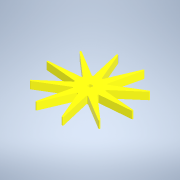
# Autodesk Inventor part: Star
Saved by Autodesk Inventor 2021 (Build 250183000, 183)
## iProperties
Created: 2021-05-22
Part Number: Star
Material: PC/ABS Plastic
Document SubType Name: Modeling
Designer: sami8
Density: 0.357273 g/cm^3
Appearance: Smooth - Yellow
Author: sami8
Autodesk Inventor part; units mm, degrees
ref_plane "YZ Plane" through (0, 0, 0) normal (1, 0, 0) x (0, 1, 0)
ref_plane "XZ Plane" through (0, 0, 0) normal (0, 1, 0) x (-1, 0, 0)
ref_plane "XY Plane" through (0, 0, 0) normal (0, 0, 1) x (1, 0, 0)
sketch "Sketch1" plane through (0, 0, 0) normal (0, 1, 0) x (-1, 0, 0)
  line L0 (2.4, -1.3856) -> (0, -2.7713)
  line L1 (0, -2.7713) -> (-2.4, -1.3856)
  line L2 (-2.4, -1.3856) -> (-2.4, 1.3856)
  line L3 (-2.4, 1.3856) -> (0, 2.7713)
  line L4 (0, 2.7713) -> (2.4, 1.3856)
  line L5 (2.4, 1.3856) -> (2.4, -1.3856)
  line L6 (0, 0) -> (2.4, 0) construction
  line L7 (0, 6) -> (70, 0)
  line L8 (70, 0) -> (0, -6)
  line L9 (0, 0) -> (0, -6)
  line L10 (0, 0) -> (0, 6)
  line L11 (0, 0) -> (70, 0) construction
  line L12 (-3.5267, 4.8541) -> (56.6312, 41.145)
  line L13 (0, 0) -> (-3.5267, 4.8541)
  line L14 (0, 0) -> (3.5267, -4.8541)
  line L15 (56.6312, 41.145) -> (3.5267, -4.8541)
  line L16 (-5.7063, 1.8541) -> (21.6312, 66.574)
  line L17 (0, 0) -> (-5.7063, 1.8541)
  line L18 (0, 0) -> (5.7063, -1.8541)
  line L19 (21.6312, 66.574) -> (5.7063, -1.8541)
  line L20 (-5.7063, -1.8541) -> (-21.6312, 66.574)
  line L21 (0, 0) -> (-5.7063, -1.8541)
  line L22 (0, 0) -> (5.7063, 1.8541)
  line L23 (-21.6312, 66.574) -> (5.7063, 1.8541)
  line L24 (-3.5267, -4.8541) -> (-56.6312, 41.145)
  line L25 (0, 0) -> (-3.5267, -4.8541)
  line L26 (0, 0) -> (3.5267, 4.8541)
  line L27 (-56.6312, 41.145) -> (3.5267, 4.8541)
  line L28 (0, -6) -> (-70, 0)
  line L29 (0, 0) -> (0, -6)
  line L30 (0, 0) -> (0, 6)
  line L31 (-70, 0) -> (0, 6)
  line L32 (3.5267, -4.8541) -> (-56.6312, -41.145)
  line L33 (0, 0) -> (3.5267, -4.8541)
  line L34 (0, 0) -> (-3.5267, 4.8541)
  line L35 (-56.6312, -41.145) -> (-3.5267, 4.8541)
  line L36 (5.7063, -1.8541) -> (-21.6312, -66.574)
  line L37 (0, 0) -> (5.7063, -1.8541)
  line L38 (0, 0) -> (-5.7063, 1.8541)
  line L39 (-21.6312, -66.574) -> (-5.7063, 1.8541)
  line L40 (5.7063, 1.8541) -> (21.6312, -66.574)
  line L41 (0, 0) -> (5.7063, 1.8541)
  line L42 (0, 0) -> (-5.7063, -1.8541)
  line L43 (21.6312, -66.574) -> (-5.7063, -1.8541)
  line L44 (3.5267, 4.8541) -> (56.6312, -41.145)
  line L45 (0, 0) -> (3.5267, 4.8541)
  line L46 (0, 0) -> (-3.5267, -4.8541)
  line L47 (56.6312, -41.145) -> (-3.5267, -4.8541)
  point P0 (14.6116, 4.7476)
  point P1 (9.0304, 12.4293)
  point P2 (0, 15.3635)
  point P3 (-9.0304, 12.4293)
  point P4 (-14.6116, 4.7476)
  point P5 (-14.6116, -4.7476)
  point P6 (-9.0304, -12.4293)
  point P7 (0, -15.3635)
  point P8 (9.0304, -12.4293)
  point P9 (14.6116, -4.7476)
  dimension "d1" = 6
  dimension "d2" = 70
  dimension "d5" = 360
  dimension "d10" = 4.8
  constraints: 96 end point, 2 collinear, 2 horizontal, 1 coincident, 1 midpoint, 1 vertical, 94 other
  measures "d1" distance of L6.start L8.end
  measures "d2" distance of L6.start L7.end
  measures "d10" distance between parallel lines of L2 L5
extrude "Extrusion1" add sketch "Sketch1" along normal blind 10 contours L5 L18 L36 L15 L14 L0 | L14 L32 L8 L9 L0 | L5 L22 L40 L19 L18 | L9 L28 L47 L25 L1 | L15 L36 L8 L32 | L5 L4 L26 L44 L23 L22 | L19 L40 L15 L36 | L25 L24 L43 L21 L2 L1 | L8 L32 L47 L28 | L10 L7 L27 L26 L4 | L3 L13 L12 L31 L10 | L3 L2 L17 L16 L35 L13 | L2 L21 L20 L39 L17 | L15 L40 L8 L36 | L8 L36 L47 L32 | L23 L44 L19 L40 | L19 L44 L15 L40 | L47 L28 L43 L24 | L47 L32 L43 L28 | L31 L12 L27 L7 | L35 L16 L31 L12 | L39 L20 L35 L16 | L43 L24 L39 L20 | L27 L7 L23 L44 | L15 L44 L8 L40 | L8 L40 L47 L36 | L47 L36 L43 L32 | L23 L7 L19 L44 | L19 L7 L15 L44 | L43 L28 L39 L24 | L43 L32 L39 L28 | L27 L12 L23 L7 | L31 L16 L27 L12 | L35 L20 L31 L16 | L39 L24 L35 L20 | L15 L7 L8 L44 | L8 L44 L47 L40 | L47 L40 L43 L36 | L43 L36 L39 L32 | L23 L12 L19 L7 | L19 L12 L15 L7 | L39 L28 L35 L24 | L39 L32 L35 L28 | L27 L16 L23 L12 | L31 L20 L27 L16 | L35 L24 L31 L20 | L23 L16 L19 L12 | L35 L28 L31 L24 | L27 L20 L23 L16 | L31 L24 L27 L20
fillet "Fillet1" radius 1 20 edges at (-70, 5, 0) (-14.6116, 5, 4.7476) (-14.6116, 5, -4.7476) (-56.6312, 5, -41.145) (-9.0304, 5, -12.4293) (-21.6312, 5, -66.574) (0, 5, -15.3635) (21.6312, 5, -66.574) (9.0304, 5, -12.4293) (56.6312, 5, -41.145) (14.6116, 5, -4.7476) (14.6116, 5, 4.7476) (9.0304, 5, 12.4293) (0, 5, 15.3635) (-9.0304, 5, 12.4293) (70, 5, 0) (56.6312, 5, 41.145) (21.6312, 5, 66.574) (-21.6312, 5, 66.574) (-56.6312, 5, 41.145)
body "Solid1"
